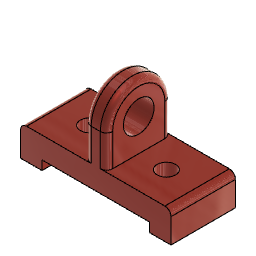
Untitled (Autodesk Fusion 360 design; units mm, degrees)
Autodesk Fusion 360 part; units mm, degrees
sketch "Sketch1" plane through (0, 0, 0) normal (0, 0, 1) x (1, 0, 0)
  line L0 (49, -21) -> (-49, -21)
  line L1 (-49, -21) -> (-49, 21)
  line L2 (-49, 21) -> (49, 21)
  line L3 (49, 21) -> (49, -21)
  line L4 (49, -21) -> (-49, 21) construction
  line L5 (-49, -21) -> (49, 21) construction
  dimension "d1" = 98
  dimension "d2" = 42
  constraint horizontal L0
  constraint perpendicular L0 L1
  constraint parallel L0 L2
  constraint parallel L1 L3
  constraint coincident L4 origin
  constraint coincident L5 origin
  measures "d1" distance of L1.end L2.end
  measures "d2" distance of L0.end L1.end
extrude "Extrude1" add sketch "Sketch1" along normal blind 20
sketch "Sketch2" plane through (0, -21, 0) normal (0, -1, 0) x (1, 0, 0)
  line L0 (-49, 0) -> (49, 0)
  line L1 (49, 0) -> (49, 20)
  line L2 (49, 20) -> (-49, 20)
  line L3 (-49, 20) -> (-49, 0)
  line L4 (-35, 0) -> (35, 0)
  line L5 (35, 0) -> (35, 6)
  line L6 (35, 6) -> (-35, 6)
  line L7 (-35, 6) -> (-35, 0)
  dimension "d5" = 6
  dimension "d6" = 14
  dimension "d7" = 14
  constraint horizontal L4
  constraint vertical L5
  constraint horizontal L6
  constraint vertical L7
  constraint coincident L0 L4.start
  measures "d5" distance of L4.start L6.end
  measures "d6" distance of L3 L7
  measures "d7" distance of L1 L5
extrude "Extrude2" cut sketch "Sketch2" against normal through all contours L0 L4 L5 L6 L7
sketch "Sketch3" plane through (0, 0, 20) normal (0, 0, 1) x (-1, 0, 0)
  line L0 (-49, -21) -> (49, -21)
  line L1 (49, -21) -> (49, 21)
  line L2 (49, 21) -> (-49, 21)
  line L3 (-49, 21) -> (-49, -21)
  line L4 (-7, 21) -> (7, 21)
  line L5 (7, 21) -> (7, -21)
  line L6 (7, -21) -> (-7, -21)
  line L7 (-7, -21) -> (-7, 21)
  line L8 (-7, 21) -> (7, -21) construction
  line L9 (7, 21) -> (-7, -21) construction
  dimension "d9" = 14
  dimension "d10" = 42
  constraint horizontal L4
  constraint perpendicular L4 L5
  constraint parallel L4 L6
  constraint parallel L5 L7
  constraint coincident L8 origin
  constraint coincident L9 origin
  measures "d9" distance of L5.end L6.end
  measures "d10" distance of L4.end L5.end
extrude "Extrude3" add sketch "Sketch3" along normal blind 42 contours L0 L2 L4 L5 L6 L7
fillet "Fillet1" radius 21 2 edges at (0, -21, 62) (0, 21, 62)
sketch "Sketch4" plane through (7, 0, 0) normal (1, 0, 0) x (0, 1, 0)
  arc A0 (21, 41) -> (-21, 41) centre (0, 41) ccw
  line L0 (-21, 41) -> (-21, 20)
  line L1 (-21, 20) -> (21, 20)
  line L2 (21, 20) -> (21, 41)
  circle A1 centre (0, 41) radius 10
  dimension "d15" = 20
  constraint concentric A0 A1
  measures "d15" diameter of A1
extrude "Extrude4" cut sketch "Sketch4" against normal through all contours A1
sketch "Sketch5" plane through (0, 0, 20) normal (0, 0, 1) x (-1, 0, 0)
  line L0 (-7, -21) -> (-7, 21)
  line L1 (-7, 21) -> (-49, 21)
  line L2 (-49, 21) -> (-49, -21)
  line L3 (-49, -21) -> (-7, -21)
  circle A0 centre (-25, 0) radius 6
  dimension "d17" = 12
  measures "d17" diameter of A0
extrude "Extrude5" cut sketch "Sketch5" against normal through all contours A0
mirror "Mirror1" about plane through (0, 0, 0) normal (1, 0, 0) of "Extrude5"
fillet "Fillet2" radius 4 8 edges at (-49, 0, 20) (-7, -21, 30.5) (-7, 0, 62) (-7, 21, 30.5) (7, -21, 30.5) (7, 0, 62) (7, 21, 30.5) (49, 0, 20)
